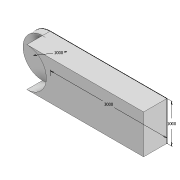
# Autodesk Inventor part: 07_LastArm
Saved by Autodesk Inventor 2022 (Build 260153000, 153)
## iProperties
Created: 2022-06-07
Part Number: 07_LastArm
Material: Generic
Document SubType Name: Modeling
Designer: pzach
Density: 1 g/cm^3
Appearance: Default
Author: pzach
Autodesk Inventor part; units mm, degrees
ref_plane "YZ Plane" through (0, 0, 0) normal (1, 0, 0) x (0, 1, 0)
ref_plane "XZ Plane" through (0, 0, 0) normal (0, 1, 0) x (-1, 0, 0)
ref_plane "XY Plane" through (0, 0, 0) normal (0, 0, 1) x (1, 0, 0)
sketch "Sketch1" plane through (0, 0, 0) normal (0, 0, 1) x (1, 0, 0)
  circle A0 centre (0, 0) radius 500
  line L0 (0, -500) -> (3000, -500)
  line L1 (3000, -500) -> (3000, 500)
  line L2 (3000, 500) -> (0, 500)
  line L3 (0, -500) -> (0, 500)
  dimension "d0" = 1000
  dimension "d1" = 3000
  dimension "d2" = 1000
  constraints: 8 end point, 2 point on circle, 2 tangent, 1 centre point, 1 coincident, 1 horizontal, 1 perpendicular
  measures "d0" diameter of A0
  measures "d1" distance of L0.start L0.end
  measures "d2" distance of L0.end L1.end
extrude "Extrusion1" add sketch "Sketch1" along normal blind 200 contours A0 L3 | L3 A0
extrude "Extrusion2" add sketch "Sketch1" along normal blind 600 contours A0 L2 L1 L0
body "Solid1"
